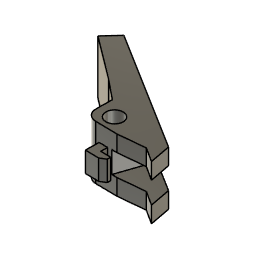
key (Autodesk Fusion 360 design; units mm, degrees)
Autodesk Fusion 360 part; units mm, degrees
note: some values were not read from the file. Chosen so that the rebuilt part matches the saved one: which face or edge a step refers to. Set by a fixed rule: which sketch regions a step uses.
sketch "Esboço1" plane through (0, 0, 0) normal (0, 0, 1) x (1, 0, 0)
  line L0 (71.5982, 50.9917) -> (71.5183, 46.0145)
  line L1 (71.5982, 50.9917) -> (65.5982, 51.0881)
  line L2 (65.5989, 51.131) -> (65.5183, 46.1108)
  line L3 (65.5183, 46.1108) -> (71.5183, 46.0145)
  line L4 (64.2741, 55.8922) -> (67.524, 51.0571)
  circle A0 centre (68.5577, 48.5402) radius 1.6
  line L5 (76.5, 46.5) -> (79.1605, 44.7883)
  line L6 (79.1605, 44.7883) -> (78.4098, 48.7074)
  line L7 (64.2741, 55.8922) -> (62, 54)
  line L8 (62, 54) -> (65.5982, 51.0881)
  line L9 (64.2741, 55.8922) -> (71.5982, 50.9917)
  line L10 (71.5183, 46.0145) -> (76.5, 46.5)
  line L11 (78.4098, 48.7074) -> (71.5982, 50.9917)
  line L12 (62, 54) -> (54, 60)
  line L13 (54, 60) -> (56.3195, 62.5072)
  line L14 (56.3195, 62.5072) -> (64.2741, 55.8922)
  line L15 (56.3195, 62.5072) -> (78.4098, 48.7074)
  dimension "d1" = 3.2
  dimension "d12" = 46.4
  dimension "d14" = 2.5
  dimension "d15" = 6
  dimension "d16" = 3
  constraint perpendicular L0 L1
  constraint perpendicular L1 L2
  constraint perpendicular L0 L3
  constraint coincident L1 L4.end
  measures "d1" diameter of A0
  measures "d12" angle of L5 L6
  measures "d14" distance of L1 A0.centre
  measures "d15" horizontal distance of L0.end L2.end
  measures "d16" distance of L2 A0.centre
extrude "Extrusão1" add sketch "Esboço1" along normal blind 10 contours L0 L5 L6 L10 L11 | L0 L1 L2 L3 | L1 L4 L9 | L1 L4 L7 L8 | L7 L12 L13 L14
fillet "Arredondamento1" radius 2 1 edges at (65.5183, 46.1108, 5)
sketch "Esboço3" plane through (22.9508, 67.526, 0) normal (0.321801, 0.946807, 0) x (-0.946807, 0.321801, 0)
  line L0 (-58.5145, 0) -> (-51.3806, 0)
  line L1 (-51.3806, 10) -> (-58.5145, 10)
  line L2 (-58.5145, 10) -> (-58.5145, 0)
  line L3 (-62.3427, 3) -> (-52, 3)
  line L4 (-52, 3) -> (-52, 7)
  line L5 (-52, 7) -> (-62.3427, 7)
  line L6 (-62.3427, 7) -> (-62.3427, 3)
  line L7 (-51.3806, 0) -> (-51.3806, 10)
  dimension "d29" = 4
  dimension "d30" = 3
  constraint horizontal L3
  constraint vertical L4
  constraint horizontal L5
  constraint vertical L6
  measures "d29" distance of L3.end L4.end
  measures "d30" distance of L0 L3
extrude "Extrusão3" cut sketch "Esboço3" against normal blind 8 contours L2 L3 L5 L6 | L2 L3 L4 L5
sketch "Esboço4" plane through (0.7573, 47.151, 0) normal (-0.016059, -0.999871, 0) x (0.999871, -0.016059, 0)
  line L0 (69.8177, 7) -> (70.7701, 7)
  line L1 (70.7701, 10) -> (66.7694, 10)
  line L2 (66.7694, 10) -> (66.7694, 0)
  line L3 (66.7694, 0) -> (70.7701, 0)
  line L4 (70.7701, 3) -> (69.8177, 3)
  line L5 (69.8177, 3) -> (69.8177, 7)
  circle A0 centre (68, 5) radius 1
  line L6 (70.7701, 7) -> (70.7701, 10)
  line L7 (70.7701, 0) -> (70.7701, 3)
scale "Escala1" factor 0.7 about (72.1847, 50.7924, 3) bodies 1
scale "Escala2" factor 1.14 about (68.5258, 49.2158, 0.9) bodies 1
extrude "Extrusão6" cut 1 faces at (76.0121, 49.8863, 4.358) along direction (0.321801, 0.946807, 0) blind 7
sketch "Esboço6" plane through (0, 0, 8.88) normal (0, 0, 1) x (-1, 0, 0)
  arc A0 (-67.4028, -48.873) -> (-68.973, -47.2516) centre (-68.9986, -48.8474) ccw
  line L0 (-68.973, -47.2516) -> (-72.1652, -47.2003)
  line L1 (-72.1652, -47.2003) -> (-76.1406, -47.5878)
  line L2 (-76.1406, -47.5878) -> (-78.2636, -46.2219)
  line L3 (-78.2636, -46.2219) -> (-77.6646, -49.3492)
  line L4 (-77.6646, -49.3492) -> (-72.229, -51.1721)
  line L5 (-72.229, -51.1721) -> (-66.3843, -55.0827)
  line L6 (-66.3843, -55.0827) -> (-60.0366, -60.3615)
  line L7 (-60.0366, -60.3615) -> (-58.1856, -58.3608)
  line L8 (-58.1856, -58.3608) -> (-64.5696, -53.5728)
  line L9 (-64.5696, -53.5728) -> (-67.441, -51.249)
  line L10 (-67.441, -51.249) -> (-67.4028, -48.873)
  circle A1 centre (-69.8026, -49.2158) radius 1.2768
  line L11 (-60.0366, -60.3615) -> (-77.6646, -49.3492)
  constraint coincident L6.end L7.start
  constraint coincident L3.end L4.start
extrude "Extrusão7" add sketch "Esboço6" against normal blind 8 contours L4 L5 L6 L11
extrude "Extrusão8" cut 1 faces at (76.0089, 49.9045, 4.358) along direction (0.31796, 0.948104, 0) blind 4.5
sketch "Esboço7" plane through (0.7765, 48.3469, 0) normal (-0.016059, -0.999871, 0) x (0.999871, -0.016059, 0)
  line L0 (71.3979, 3.294) -> (70.6379, 3.294)
  line L1 (70.6379, 3.294) -> (70.6379, 6.486)
  line L2 (70.6379, 6.486) -> (71.3979, 6.486)
  line L3 (71.3979, 6.486) -> (71.3979, 8.88)
  line L4 (71.3979, 8.88) -> (68.2053, 8.88)
  line L5 (68.2053, 8.88) -> (68.2053, 0.9)
  line L6 (68.2053, 0.9) -> (71.3979, 0.9)
  line L7 (71.3979, 0.9) -> (71.3979, 3.294)
  line L8 (68.7249, 6.435) -> (70, 6.435)
  line L9 (70, 6.435) -> (70, 3.435)
  line L10 (70, 3.435) -> (68.7249, 3.435)
  line L11 (68.7249, 3.435) -> (68.7249, 6.435)
  dimension "d47" = 3
  constraint horizontal L8
  constraint vertical L9
  constraint horizontal L10
  constraint vertical L11
  measures "d47" distance of L8.start L10.end
extrude "Extrusão9" add sketch "Esboço7" along normal blind 2 contours L8 L9 L10 L11
sketch "Esboço8" plane through (69.991, -1.1241, 0) normal (0.999871, -0.016059, 0) x (0.016059, 0.999871, 0)
  line L0 (48.3531, 3.435) -> (48.3531, 6.435)
  line L1 (48.3531, 6.435) -> (46.3531, 6.435)
  line L2 (46.3531, 6.435) -> (46.3531, 3.435)
  line L3 (46.3531, 3.435) -> (48.3531, 3.435)
  line L4 (46.3531, 6.435) -> (47.3531, 6.435)
  line L5 (47.3531, 6.435) -> (47.3531, 3.435)
  line L6 (47.3531, 3.435) -> (46.3531, 3.435)
  line L7 (46.3531, 3.435) -> (46.3531, 6.435)
  constraint horizontal L4
  constraint vertical L5
  constraint horizontal L6
  constraint vertical L7
  constraint midpoint L3 L5.end
  constraint coincident L1.end L2.start
extrude "Extrusão10" add sketch "Esboço8" along normal blind 1.5 contours L1 L2 L3 L4 L5 L6 L7
sketch "Esboço9" plane through (0, 0, 6.435) normal (0, 0, 1) x (-1, 0, 0)
  line L0 (-70.7675, -47.2228) -> (-69.4925, -47.2432)
  line L1 (-69.4925, -47.2432) -> (-69.4604, -45.2435)
  line L2 (-69.4604, -45.2435) -> (-72.2352, -45.1989)
  line L3 (-72.2352, -45.1989) -> (-72.2512, -46.1988)
  line L4 (-72.2512, -46.1988) -> (-70.7514, -46.2229)
  line L5 (-70.7514, -46.2229) -> (-70.7675, -47.2228)
  line L6 (-71.4473, -45.2116) -> (-72.2432, -45.6989)
  constraint midpoint L3 L6.end
  constraint coincident L2 L6.start
extrude "Extrusão11" cut sketch "Esboço9" against normal blind 3.3 contours L2 L3 L6
